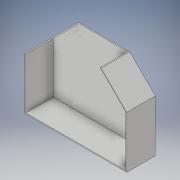
# Autodesk Inventor part: 15102898-16-P-0203
Saved by Autodesk Inventor 2017 (Build 210142000, 142)
## iProperties
Created: 2016-10-01
Part Number: 15102898-16-P-0203
Material: Generic
Document SubType Name: Modeling
Designer: Sofia
Density: 1 g/cm^3
Appearance: Default
Author: Sofia
Autodesk Inventor part; units mm, degrees
ref_plane "YZ Plane" through (0, 0, 0) normal (1, 0, 0) x (0, 1, 0)
ref_plane "XZ Plane" through (0, 0, 0) normal (0, 1, 0) x (-1, 0, 0)
ref_plane "XY Plane" through (0, 0, 0) normal (0, 0, 1) x (1, 0, 0)
sketch "Sketch1" plane through (0, 0, 0) normal (0, 1, 0) x (-1, 0, 0)
  line L0 (0, 0) -> (-304.8, 0)
  line L1 (-304.8, 0) -> (-304.8, -84.8294)
  line L2 (-304.8, -84.8294) -> (0, -84.8294)
  line L3 (0, -84.8294) -> (0, 0)
  dimension "d0" = 304.8
  constraints: 8 end point, 2 parallel, 1 horizontal, 1 perpendicular
  measures "d0" distance of L2.end L1.end
extrude "Extrusion1" add sketch "Sketch1" along normal blind 3.175
sketch "Sketch2" plane through (0, 3.175, 0) normal (0, 1, 0) x (1, 0, 0)
  line L0 (0, 0) -> (304.8, 0) projected
  line L1 (3.175, 0) -> (3.175, 81.6544)
  line L2 (3.175, 81.6544) -> (301.625, 81.6544)
  line L3 (301.625, 81.6544) -> (301.625, 0)
  line L4 (304.8, 0) -> (304.8, 84.8294) projected
  line L5 (0, 84.8294) -> (0, 0) projected
  line L6 (304.8, 84.8294) -> (0, 84.8294) projected
  line L7 (0, 0) -> (3.175, 0)
  line L8 (304.8, 0) -> (301.625, 0)
  dimension "d3" = 3.175
  dimension "d4" = 3.175
  dimension "d5" = 3.175
  constraints: 10 end point, 2 collinear, 2 perpendicular, 1 point on line, 1 vertical
  measures "d3" distance between parallel lines of L4 L3
  measures "d4" distance between parallel lines of L1 L5
  measures "d5" distance between parallel lines of L6 L2
extrude "Extrusion2" add sketch "Sketch2" along normal blind 152.4 contours L5 L6 L4 L0 L3 L2 L1
sketch "Sketch4" plane through (3.175, 3.175, -81.6544) normal (0, 0, 1) x (1, 0, 0)
  line L0 (-3.175, 152.4) -> (73.025, 228.6)
  line L1 (301.625, 152.4) -> (-3.175, 152.4) projected
  line L2 (301.625, 152.4) -> (225.425, 228.6)
  line L3 (225.425, 228.6) -> (73.025, 228.6)
  point P0 (-3.175, -3.175)
  point P1 (-3.175, 152.4)
  dimension "d11" = 152.4
  dimension "d12" = 76.2
  constraints: 6 end point, 1 coincident, 1 parallel, 1 perpendicular
  measures "d11" distance of L2.end L0.end
  measures "d12" distance between parallel lines of L1 L3
extrude "Extrusion3" add sketch "Sketch4" against normal blind 3.175
sketch "Sketch7" plane through (3.175, 3.175, -81.6544) normal (0, 0, 1) x (1, 0, 0)
  line L0 (0.6738, 152.4) -> (76.8738, 228.6)
  line L1 (-3.175, 152.4) -> (73.025, 228.6) projected
  line L2 (0.6738, 152.4) -> (-3.175, 152.4)
  line L3 (73.025, 228.6) -> (225.425, 228.6) projected
  line L4 (73.025, 228.6) -> (76.8738, 228.6)
  point P0 (-3.175, -3.175)
  constraints: 6 end point, 1 collinear, 1 horizontal, 1 parallel
extrude "Extrusion4" add sketch "Sketch7" along normal blind 82.042
sketch "Sketch8" plane through (3.175, 3.175, -81.6544) normal (0, 0, 1) x (1, 0, 0)
  line L0 (301.625, -3.175) -> (301.625, 152.4) projected
  line L1 (298.45, 0) -> (298.45, 152.4) projected
  line L2 (301.625, 152.4) -> (298.45, 152.4)
  line L3 (298.45, 152.4) -> (222.25, 228.6)
  line L4 (76.8738, 228.6) -> (225.425, 228.6) projected
  line L5 (301.625, 152.4) -> (225.425, 228.6)
  point P0 (-3.175, -3.175)
  dimension "d19" = 3.175
  constraints: 6 end point, 1 horizontal, 1 point on line
  measures "d19" distance of L4.end L3.end
extrude "Extrusion5" add sketch "Sketch8" along normal blind 82.042
body "Solid1"
